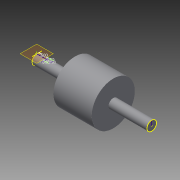
# Autodesk Inventor part: Ring1_Roller_JacobMorgan_030315_pd3
Saved by Autodesk Inventor 2015 (Build 190159000, 159)
## iProperties
Created: 2015-03-03
Part Number: Ring1_Roller_JacobMorgan_030315_pd3
Material: Generic
Document SubType Name: Modeling
Designer: WASHHSST
Density: 1 g/cm^3
Appearance: Default
Author: WASHHSST
Autodesk Inventor part; units mm, degrees
ref_plane "YZ Plane" through (0, 0, 0) normal (1, 0, 0) x (0, 1, 0)
ref_plane "XZ Plane" through (0, 0, 0) normal (0, 1, 0) x (-1, 0, 0)
ref_plane "XY Plane" through (0, 0, 0) normal (0, 0, 1) x (1, 0, 0)
sketch "Sketch3" plane through (0, 0, 0) normal (1, 0, 0) x (0, 1, 0)
  circle A0 centre (0, 0) radius 28.575
  dimension "d11" = 57.15
  constraints: 1 centre point, 1 coincident
  measures "d11" diameter of A0
extrude "Extrusion3" add sketch "Sketch3" along normal blind 50.8
sketch "Sketch4" plane through (50.8, 0, 0) normal (1, 0, 0) x (0, 0, -1)
  circle A0 centre (0, 0) radius 6.35
  dimension "d14" = 12.7
  constraints: 1 centre point, 1 coincident
  measures "d14" diameter of A0
sketch "Sketch5" plane through (0, 0, 0) normal (-1, 0, 0) x (0, 0, 1)
  circle A0 centre (0, 0) radius 6.35
  dimension "d15" = 12.7
  constraints: 1 centre point, 1 coincident
  measures "d15" diameter of A0
extrude "Extrusion4" add sketch "Sketch5" along normal blind 50.8
extrude "Extrusion5" add sketch "Sketch4" along normal blind 50.8
sketch "Sketch6" plane through (101.6, 0, 0) normal (1, 0, 0) x (0, 0, -1)
  line L0 (0, 0) -> (0, 6.35)
  circle A0 centre (0, 0) radius 6.35 projected
  constraints: 2 end point, 1 vertical, 1 vertical alignment, 1 other
sketch "Sketch7" plane through (-50.8, 0, 0) normal (-1, 0, 0) x (0, 0, 1)
  line L0 (0, 0) -> (0, 6.35)
  circle A0 centre (0, 0) radius 6.35 projected
  constraints: 2 end point, 1 vertical, 1 vertical alignment, 1 other
sketch "Sketch8" plane through (-50.8, 0, 0) normal (-1, 0, 0) x (0, 0, 1)
  circle A0 centre (0, 0) radius 6.35 projected
  point P0 (0, 6.35)
  constraints: 1 vertical alignment, 1 other
ref_plane "Work Plane1" through (-50.8, 6.35, 0) normal (0, 1, 0) x (-1, 0, 0)
sketch "Sketch9" plane through (-50.8, 6.35, 0) normal (0, 1, 0) x (-1, 0, 0)
  line L0 (0, -6.35) -> (0, 6.35) projected
  line L1 (0, 0) -> (-12.7, 0)
  line L2 (-12.7, 0) -> (-12.7, 6.35)
  line L3 (-12.7, 0) -> (-12.7, 3.175)
  line L4 (-12.7, 3.175) -> (-19.05, 3.175)
  line L5 (-19.05, 3.175) -> (-19.05, -3.175)
  line L6 (-19.05, -3.175) -> (-12.7, -3.175)
  line L7 (-12.7, -3.175) -> (-12.7, 3.175)
  point P0 (-50.8, 0)
  dimension "d20" = 12.7
  dimension "d21" = 6.35
  dimension "d23" = 6.35
  dimension "d24" = 6.35
  dimension "d26" = 6.35
  constraints: 14 end point, 2 horizontal, 2 midpoint, 2 perpendicular, 1 vertical
  measures "d20" distance of L1.start L1.end
  measures "d21" distance of L1.end L2.end
  measures "d23" distance of L3.end L4.end
  measures "d24" distance of L4.end L5.end
  measures "d26" distance of L5.end L6.end
body "Solid2"
